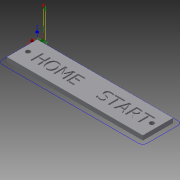
# Autodesk Inventor part: label
Saved by Autodesk Inventor 2015 SP1 (Build 190203100, 203)
## iProperties
Created: 2015-08-11
Part Number: label
Material: Generic
Document SubType Name: Modeling
Designer: ubik
Density: 1 g/cm^3
Appearance: Default
Author: ubik
Autodesk Inventor part; units mm, degrees
ref_plane "YZ Plane" through (0, 0, 0) normal (1, 0, 0) x (0, 1, 0)
ref_plane "XZ Plane" through (0, 0, 0) normal (0, 1, 0) x (-1, 0, 0)
ref_plane "XY Plane" through (0, 0, 0) normal (0, 0, 1) x (1, 0, 0)
sketch "Sketch1" plane through (0, 0, 0) normal (0, 0, 1) x (1, 0, 0)
  line L0 (-45, 10) -> (45, 10)
  line L1 (45, 10) -> (45, -10)
  line L2 (45, -10) -> (-45, -10)
  line L3 (-45, -10) -> (-45, 10)
  point P0 (0, 0)
  dimension "d0" = 90
  dimension "d1" = 20
  dimension "d2" = 10
  dimension "d3" = 45
  constraints: 8 end point, 2 parallel, 1 horizontal, 1 perpendicular
  measures "d0" distance of L1.end L2.end
  measures "d1" distance of L0.end L1.end
  measures "d2" distance from line of point (0, 0) L0
  measures "d3" distance from line of point (0, 0) L3
extrude "Extrusion1" add sketch "Sketch1" along normal blind 3
sketch "Sketch2" plane through (0, 0, 3) normal (0, 0, 1) x (1, 0, 0)
  line L0 (-36.2796, 4.097) -> (-23.2127, 4.097) construction
  line L1 (-23.2127, 4.097) -> (-23.2127, 0.4495) construction
  line L2 (-23.2127, 0.4495) -> (-36.2796, 0.4495) construction
  line L3 (-36.2796, 0.4495) -> (-36.2796, 4.097) construction
  line L4 (6.7486, 4.3702) -> (20.9273, 4.3702) construction
  line L5 (20.9273, 4.3702) -> (20.9273, 0.7454) construction
  line L6 (20.9273, 0.7454) -> (6.7486, 0.7454) construction
  line L7 (6.7486, 0.7454) -> (6.7486, 4.3702) construction
  spline S0 degree 2 poles (9.7891, -3.9151) (8.9204, -3.9151) (7.7016, -3.552) (7.1635, -3.2927) knots 0 0 0 1 2 2 2
  line L8 (7.1635, -3.2927) -> (7.1635, -1.9572)
  line L9 (7.1635, -1.9572) -> (7.2413, -1.9572)
  spline S1 degree 2 poles (7.2413, -1.9572) (7.7664, -2.4499) (9.0954, -2.9945) (9.7113, -2.9945) knots 0 0 0 1 2 2 2
  spline S2 degree 2 poles (9.7113, -2.9945) (10.593, -2.9945) (11.4941, -2.2619) (11.4941, -1.659) knots 0 0 0 1 2 2 2
  spline S3 degree 2 poles (11.4941, -1.659) (11.4941, -1.1793) (11.0209, -0.5828) (10.5087, -0.4337) knots 0 0 0 1 2 2 2
  spline S4 degree 2 poles (10.5087, -0.4337) (10.1392, -0.33) (9.5233, -0.1874) (9.063, -0.0707) knots 0 0 0 1 2 2 2
  spline S5 degree 2 poles (9.063, -0.0707) (8.6481, 0.0395) (7.9933, 0.3702) (7.7405, 0.636) knots 0 0 0 1 2 2 2
  spline S6 degree 2 poles (7.7405, 0.636) (7.4941, 0.9018) (7.2218, 1.6149) (7.2218, 2.0817) knots 0 0 0 1 2 2 2
  spline S7 degree 2 poles (7.2218, 2.0817) (7.2218, 3.0541) (8.7389, 4.3702) (9.9123, 4.3702) knots 0 0 0 1 2 2 2
  spline S8 degree 2 poles (9.9123, 4.3702) (10.5865, 4.3702) (11.7794, 4.1044) (12.2915, 3.8515) knots 0 0 0 1 2 2 2
  line L10 (12.2915, 3.8515) -> (12.2915, 2.5809)
  line L11 (12.2915, 2.5809) -> (12.2137, 2.5809)
  spline S9 degree 2 poles (12.2137, 2.5809) (11.8312, 2.9309) (10.6384, 3.4496) (9.9836, 3.4496) knots 0 0 0 1 2 2 2
  spline S10 degree 2 poles (9.9836, 3.4496) (9.2445, 3.4496) (8.3304, 2.7559) (8.3304, 2.1919) knots 0 0 0 1 2 2 2
  spline S11 degree 2 poles (8.3304, 2.1919) (8.3304, 1.6862) (8.8685, 1.0833) (9.3742, 0.9471) knots 0 0 0 1 2 2 2
  spline S12 degree 2 poles (9.3742, 0.9471) (9.7113, 0.8564) (10.6902, 0.623) (11.0144, 0.5258) knots 0 0 0 1 2 2 2
  spline S13 degree 2 poles (11.0144, 0.5258) (11.8377, 0.2729) (12.6027, -0.7449) (12.6027, -1.4905) knots 0 0 0 1 2 2 2
  spline S14 degree 2 poles (12.6027, -1.4905) (12.6027, -1.9637) (12.2202, -2.8713) (11.8766, -3.189) knots 0 0 0 1 2 2 2
  spline S15 degree 2 poles (11.8766, -3.189) (11.4941, -3.5391) (10.5217, -3.9151) (9.7891, -3.9151) knots 0 0 0 1 2 2 2
  line L12 (15.5525, -3.7725) -> (15.5525, 3.281)
  line L13 (15.5525, 3.281) -> (12.8685, 3.281)
  line L14 (12.8685, 3.281) -> (12.8685, 4.2275)
  line L15 (12.8685, 4.2275) -> (19.2996, 4.2275)
  line L16 (19.2996, 4.2275) -> (19.2996, 3.281)
  line L17 (19.2996, 3.281) -> (16.6157, 3.281)
  line L18 (16.6157, 3.281) -> (16.6157, -3.7725)
  line L19 (16.6157, -3.7725) -> (15.5525, -3.7725)
  line L20 (19.2478, -3.7725) -> (21.9447, 4.2275)
  line L21 (21.9447, 4.2275) -> (23.2543, 4.2275)
  line L22 (23.2543, 4.2275) -> (25.9512, -3.7725)
  line L23 (25.9512, -3.7725) -> (24.8296, -3.7725)
  line L24 (24.8296, -3.7725) -> (24.1035, -1.5358)
  line L25 (24.1035, -1.5358) -> (21.05, -1.5358)
  line L26 (21.05, -1.5358) -> (20.3239, -3.7725)
  line L27 (20.3239, -3.7725) -> (19.2478, -3.7725)
  line L28 (23.8118, -0.6282) -> (22.5735, 3.1384)
  line L29 (22.5735, 3.1384) -> (21.3418, -0.6282)
  line L30 (21.3418, -0.6282) -> (23.8118, -0.6282)
  line L31 (32.9009, -3.7725) -> (31.5201, -3.7725)
  line L32 (31.5201, -3.7725) -> (28.9917, -0.5893)
  line L33 (28.9917, -0.5893) -> (27.7729, -0.5893)
  line L34 (27.7729, -0.5893) -> (27.7729, -3.7725)
  line L35 (27.7729, -3.7725) -> (26.7097, -3.7725)
  line L36 (26.7097, -3.7725) -> (26.7097, 4.2275)
  line L37 (26.7097, 4.2275) -> (28.7713, 4.2275)
  spline S16 degree 2 poles (28.7713, 4.2275) (29.4585, 4.2275) (30.3855, 4.0784) (30.8069, 3.8061) knots 0 0 0 1 2 2 2
  spline S17 degree 2 poles (30.8069, 3.8061) (31.2283, 3.5339) (31.7145, 2.6846) (31.7145, 2.0557) knots 0 0 0 1 2 2 2
  spline S18 degree 2 poles (31.7145, 2.0557) (31.7145, 1.1805) (30.8199, -0.0058) (30.0549, -0.2911) knots 0 0 0 1 2 2 2
  line L38 (30.0549, -0.2911) -> (32.9009, -3.7725)
  spline S19 degree 2 poles (30.606, 1.9715) (30.606, 2.3215) (30.3596, 2.8596) (30.1003, 3.0347) knots 0 0 0 1 2 2 2
  spline S20 degree 2 poles (30.1003, 3.0347) (29.8734, 3.1838) (29.2705, 3.307) (28.8296, 3.307) knots 0 0 0 1 2 2 2
  line L39 (28.8296, 3.307) -> (27.7729, 3.307)
  line L40 (27.7729, 3.307) -> (27.7729, 0.2989)
  line L41 (27.7729, 0.2989) -> (28.7064, 0.2989)
  spline S21 degree 2 poles (28.7064, 0.2989) (29.1667, 0.2989) (29.8993, 0.4609) (30.1522, 0.7138) knots 0 0 0 1 2 2 2
  spline S22 degree 2 poles (30.1522, 0.7138) (30.3855, 0.9342) (30.606, 1.5565) (30.606, 1.9715) knots 0 0 0 1 2 2 2
  line L42 (35.4034, -3.7725) -> (35.4034, 3.281)
  line L43 (35.4034, 3.281) -> (32.7194, 3.281)
  line L44 (32.7194, 3.281) -> (32.7194, 4.2275)
  line L45 (32.7194, 4.2275) -> (39.1505, 4.2275)
  line L46 (39.1505, 4.2275) -> (39.1505, 3.281)
  line L47 (39.1505, 3.281) -> (36.4666, 3.281)
  line L48 (36.4666, 3.281) -> (36.4666, -3.7725)
  line L49 (36.4666, -3.7725) -> (35.4034, -3.7725)
  line L50 (-29.6604, -4.0716) -> (-30.7237, -4.0716)
  line L51 (-30.7237, -4.0716) -> (-30.7237, -0.1558)
  line L52 (-30.7237, -0.1558) -> (-34.406, -0.1558)
  line L53 (-34.406, -0.1558) -> (-34.406, -4.0716)
  line L54 (-34.406, -4.0716) -> (-35.4692, -4.0716)
  line L55 (-35.4692, -4.0716) -> (-35.4692, 3.9284)
  line L56 (-35.4692, 3.9284) -> (-34.406, 3.9284)
  line L57 (-34.406, 3.9284) -> (-34.406, 0.7907)
  line L58 (-34.406, 0.7907) -> (-30.7237, 0.7907)
  line L59 (-30.7237, 0.7907) -> (-30.7237, 3.9284)
  line L60 (-30.7237, 3.9284) -> (-29.6604, 3.9284)
  line L61 (-29.6604, 3.9284) -> (-29.6604, -4.0716)
  spline S23 degree 2 poles (-22.3801, 3.0143) (-21.9262, 2.4827) (-21.4206, 0.9268) (-21.4206, -0.0716) knots 0 0 0 1 2 2 2
  spline S24 degree 2 poles (-21.4206, -0.0716) (-21.4206, -1.044) (-21.9133, -2.6194) (-22.3801, -3.151) knots 0 0 0 1 2 2 2
  spline S25 degree 2 poles (-22.3801, -3.151) (-22.8728, -3.7085) (-24.1758, -4.2401) (-24.9603, -4.2401) knots 0 0 0 1 2 2 2
  spline S26 degree 2 poles (-24.9603, -4.2401) (-25.7707, -4.2401) (-27.0673, -3.6891) (-27.5405, -3.151) knots 0 0 0 1 2 2 2
  spline S27 degree 2 poles (-27.5405, -3.151) (-28.0008, -2.6194) (-28.4935, -1.057) (-28.4935, -0.0716) knots 0 0 0 1 2 2 2
  spline S28 degree 2 poles (-28.4935, -0.0716) (-28.4935, 0.9333) (-27.9943, 2.4633) (-27.534, 3.0143) knots 0 0 0 1 2 2 2
  spline S29 degree 2 poles (-27.534, 3.0143) (-27.0673, 3.546) (-25.7642, 4.097) (-24.9603, 4.097) knots 0 0 0 1 2 2 2
  spline S30 degree 2 poles (-24.9603, 4.097) (-24.1434, 4.097) (-22.8339, 3.5265) (-22.3801, 3.0143) knots 0 0 0 1 2 2 2
  spline S31 degree 2 poles (-22.5292, -0.0716) (-22.5292, 0.7194) (-22.8728, 1.9447) (-23.1839, 2.3466) knots 0 0 0 1 2 2 2
  spline S32 degree 2 poles (-23.1839, 2.3466) (-23.5016, 2.7615) (-24.3963, 3.1764) (-24.9538, 3.1764) knots 0 0 0 1 2 2 2
  spline S33 degree 2 poles (-24.9538, 3.1764) (-25.5308, 3.1764) (-26.3995, 2.7745) (-26.7301, 2.3466) knots 0 0 0 1 2 2 2
  spline S34 degree 2 poles (-26.7301, 2.3466) (-27.0478, 1.9382) (-27.3849, 0.7064) (-27.3849, -0.0716) knots 0 0 0 1 2 2 2
  spline S35 degree 2 poles (-27.3849, -0.0716) (-27.3849, -1.6469) (-26.0624, -3.3195) (-24.9538, -3.3195) knots 0 0 0 1 2 2 2
  spline S36 degree 2 poles (-24.9538, -3.3195) (-23.8452, -3.3195) (-22.5292, -1.6469) (-22.5292, -0.0716) knots 0 0 0 1 2 2 2
  line L62 (-13.3946, -4.0716) -> (-14.4579, -4.0716)
  line L63 (-14.4579, -4.0716) -> (-14.4579, 2.8199)
  line L64 (-14.4579, 2.8199) -> (-16.5454, -1.8673)
  line L65 (-16.5454, -1.8673) -> (-17.1937, -1.8673)
  line L66 (-17.1937, -1.8673) -> (-19.2617, 2.8199)
  line L67 (-19.2617, 2.8199) -> (-19.2617, -4.0716)
  line L68 (-19.2617, -4.0716) -> (-20.2536, -4.0716)
  line L69 (-20.2536, -4.0716) -> (-20.2536, 3.9284)
  line L70 (-20.2536, 3.9284) -> (-18.8015, 3.9284)
  line L71 (-18.8015, 3.9284) -> (-16.8047, -0.5254)
  line L72 (-16.8047, -0.5254) -> (-14.8728, 3.9284)
  line L73 (-14.8728, 3.9284) -> (-13.3946, 3.9284)
  line L74 (-13.3946, 3.9284) -> (-13.3946, -4.0716)
  line L75 (-11.7739, -4.0716) -> (-11.7739, 3.9284)
  line L76 (-11.7739, 3.9284) -> (-6.769, 3.9284)
  line L77 (-6.769, 3.9284) -> (-6.769, 2.9819)
  line L78 (-6.769, 2.9819) -> (-10.7107, 2.9819)
  line L79 (-10.7107, 2.9819) -> (-10.7107, 0.7907)
  line L80 (-10.7107, 0.7907) -> (-7.0348, 0.7907)
  line L81 (-7.0348, 0.7907) -> (-7.0348, -0.1558)
  line L82 (-7.0348, -0.1558) -> (-10.7107, -0.1558)
  line L83 (-10.7107, -0.1558) -> (-10.7107, -3.125)
  line L84 (-10.7107, -3.125) -> (-6.769, -3.125)
  line L85 (-6.769, -3.125) -> (-6.769, -4.0716)
  line L86 (-6.769, -4.0716) -> (-11.7739, -4.0716)
  point P0 (0, 0)
  constraints: 4 other
extrude "Extrusion2" cut sketch "Sketch2" against normal blind 1
hole "Hole1" at (-41, 0, 3) direction (0, 0, -1) diameter 3 end through all
hole "Hole2" at (41, 0, 3) direction (0, 0, -1) diameter 3 end through all
equation "\"d2\" = 0.5 * d1"
equation "\"d3\" = 0.5 * d0"
body "Solid1"
